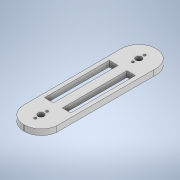
# Autodesk Inventor part: new arm
Saved by Autodesk Inventor 2022 (Build 260153000, 153)
## iProperties
Created: 2021-06-21
Part Number: new arm
Material: Generic
Document SubType Name: Sheet Metal
Designer: mohammed
Density: 1 g/cm^3
Sheet Metal Rule: Default
Appearance: Default
Author: mohammed
Autodesk Inventor part; units mm, degrees
ref_plane "YZ Plane" through (0, 0, 0) normal (1, 0, 0) x (0, 1, 0)
ref_plane "XZ Plane" through (0, 0, 0) normal (0, 1, 0) x (-1, 0, 0)
ref_plane "XY Plane" through (0, 0, 0) normal (0, 0, 1) x (1, 0, 0)
sketch "Sketch1" plane through (0, 0, 0) normal (0, 1, 0) x (-1, 0, 0)
  circle A0 centre (-34.9394, -164.0528) radius 94.5846
  circle A1 centre (-34.4972, 20.1632) radius 38.5234
  circle A2 centre (-34.4972, -347.6177) radius 38.24
  line L0 (-41.6734, 3421.2475) -> (-14.4978, 3421.2475)
  line L1 (-118.1258, -698.8711) -> (48.2471, -698.8711)
  line L2 (-571.1236, 2945.3673) -> (-571.1236, -90.1812)
  line L3 (505.8676, 2926.6588) -> (505.8676, -185.9236)
  circle A3 centre (-28.0856, 2885.9144) radius 94.5846
  circle A4 centre (-32.9097, 3069.0726) radius 38.5234
  circle A5 centre (-32.9097, 2701.2918) radius 38.24
  arc A6 (505.8676, 2845.1699) -> (-41.6734, 3421.2475) centre (-28.0856, 2885.9144) ccw
  arc A7 (-571.1236, -90.1812) -> (505.8676, -142.1821) centre (-34.9394, -164.0528) ccw
  arc A8 (-41.6734, 3421.2475) -> (-571.1236, 2945.3673) centre (-41.6734, 2888.782) ccw
  line L4 (-571.1236, 2371.0918) -> (505.8676, 2371.0918)
  line L5 (-571.1236, 350.3632) -> (505.8676, 350.3632)
  line L6 (-444.1236, 2371.0918) -> (-444.1236, 350.3632)
  line L7 (99.4676, 2371.0918) -> (99.4676, 350.3632)
  line L8 (378.8676, 2371.0918) -> (378.8676, 350.3632)
  line L9 (-32.628, 2371.0918) -> (-32.628, 2350.4281)
  line L10 (-32.628, 377.1913) -> (-32.628, 350.3632)
  line L11 (-179.9324, 2371.0918) -> (-179.9324, 350.3632)
  point P0 (0, 0)
  point P1 (-40.1425, -163.2624)
  dimension "d0" = 535.5055
  dimension "d1" = 189.1691
  dimension "d2" = 76.48
  dimension "d3" = 77.0468
  dimension "d4" = 541.2491
  dimension "d5" = 532.4654
  dimension "d6" = 1076.9912
  dimension "d7" = 505.8676
  dimension "d8" = 457.6205
  dimension "d9" = 520.3654
  dimension "d10" = 533.9532
  dimension "d11" = 538.7773
  dimension "d12" = 538.7773
  dimension "d13" = 540.3648
  dimension "d14" = 540.3648
  dimension "d15" = 540.807
  dimension "d16" = 700.5345
  dimension "d17" = 39.9576
  dimension "d18" = 349.3252
  dimension "d19" = 2970.0562
  dimension "d20" = 3069.2491
  dimension "d21" = 2701.4922
  dimension "d22" = 546.0101
  dimension "d23" = 535.6087
  dimension "d24" = 330.2
  dimension "d25" = 330.2
  dimension "d26" = 127
  dimension "d27" = 279.4
  dimension "d28" = 127
  dimension "d29" = 279.4
  constraints: 24 end point, 14 point on line, 13 point on circle, 9 centre point, 5 perpendicular, 3 equal radius, 2 coincident, 2 horizontal, 2 midpoint, 2 parallel, 2 vertical, 1 tangent
  measures "d0" radius of A6
  measures "d1" diameter of A3
  measures "d2" diameter of A5
  measures "d3" diameter of A1
  measures "d4" radius of A7
  measures "d5" radius of A8
  measures "d6" distance between parallel lines of L2 L3
  measures "d7" distance from line of point (0, 0) L3
  measures "d8" distance from line of L1.end L3
  measures "d9" distance from line of L0.end L3
  measures "d10" distance from line of A6.centre L3
  measures "d11" distance from line of A4.centre L3
  measures "d12" distance from line of A5.centre L3
  measures "d13" distance from line of A1.centre L3
  measures "d14" distance from line of A2.centre L3
  measures "d15" distance from line of A0.centre L3
  measures "d16" distance of point (0, 0) L1.end
  measures "d17" distance of point (0, 0) A1.centre
  measures "d18" distance of point (0, 0) A2.centre
  measures "d19" distance of L3.start point (0, 0)
  measures "d20" distance of A4.centre point (0, 0)
  measures "d21" distance of A5.centre point (0, 0)
  measures "d22" distance from line of point (-40.143, -163.262) L3
  measures "d23" distance from line of point (-40.143, -163.262) L1
  measures "d24" distance from line of L4 A5.centre
  measures "d25" distance from line of L5 A1.centre
  measures "d26" distance between parallel lines of L3 L8
  measures "d27" distance between parallel lines of L8 L7
  measures "d28" distance between parallel lines of L2 L6
  measures "d29" distance between parallel lines of L7 L11
extrude "Extrusion1" add sketch "Sketch1" along normal blind 177.8 contours L0 A6 L3 L4 L2 A8 | L4 L6 L5 L2 | L5 L3 A7 L1 L2 | L3 L5 L8 L4 | L4 L7 L5 L11
equation "\"BendRadius\" = Thickness"
equation "\"BendReliefWidth\" = Thickness"
equation "\"BendReliefDepth\" = 0.5 * Thickness"
equation "\"CornerReliefSize\" = 4 * Thickness"
equation "\"MinimumRemnant\" = 2 * Thickness"
equation "\"TransitionRadius\" = BendRadius"
equation "\"JacobiRadiusSize\" = BendRadius"
equation "\"GapSize\" = Thickness"
equation "\"Thickness\" = 3.048"
body "Solid1"
